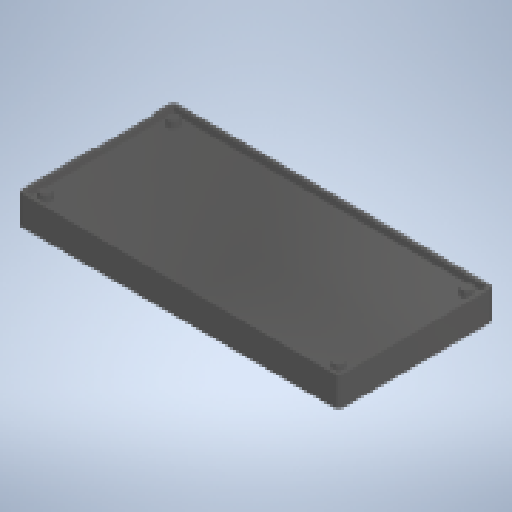
# Autodesk Inventor part: base
Saved by Autodesk Inventor 2025.3 (Build 293356000, 356)
## iProperties
Created: 2025-05-23
Part Number: base
Material: Generic
Document SubType Name: Modeling
Designer: Yuhsuan Chen
Density: 1 g/cm^3
Appearance: Default
Author: Yuhsuan Chen
Autodesk Inventor part; units mm, degrees
ref_plane "YZ Plane" through (0, 0, 0) normal (1, 0, 0) x (0, 1, 0)
ref_plane "XZ Plane" through (0, 0, 0) normal (0, 1, 0) x (-1, 0, 0)
ref_plane "XY Plane" through (0, 0, 0) normal (0, 0, 1) x (1, 0, 0)
sketch "Sketch1" plane through (0, 0, 0) normal (0, 1, 0) x (-1, 0, 0)
  line L0 (0, 20) -> (-92, 20)
  line L1 (-92, 20) -> (-92, -20)
  line L2 (-92, -20) -> (0, -20)
  line L3 (0, -20) -> (0, 20)
  line L4 (-46, 20) -> (-46, -20) construction
  line L5 (0, 0) -> (-92, 0) construction
  line L6 (0.15, 20.15) -> (-92.15, 20.15)
  line L7 (-92.15, 20.15) -> (-92.15, -20.15)
  line L8 (-92.15, -20.15) -> (0.15, -20.15)
  line L9 (0.15, -20.15) -> (0.15, 20.15)
  dimension "d0" = 40
  dimension "d1" = 92
  dimension "d19" = 0.15
  constraints: 20 end point, 4 midpoint, 4 parallel, 2 coincident, 2 perpendicular, 1 horizontal, 3 other
  measures "d0" distance of L2.end L0.start
  measures "d1" distance of L0.start L0.end
  measures "d19" distance between parallel lines of L3 L9
extrude "Extrusion1" add sketch "Sketch1" along normal blind 0.7 contours L3 L2 L1 L0 | L9 L8 L7 L6
sketch "Sketch2" plane through (0, 0.7, 0) normal (0, 1, 0) x (1, 0, 0)
  line L0 (92.15, -20.15) -> (92.15, 20.15) projected
  line L1 (92.15, 20.15) -> (-0.15, 20.15) projected
  line L2 (-0.15, 20.15) -> (-0.15, -20.15) projected
  line L3 (-0.15, -20.15) -> (92.15, -20.15) projected
  line L4 (1.05, -18.95) -> (1.05, 18.95)
  line L5 (1.05, 18.95) -> (90.95, 18.95)
  line L6 (90.95, 18.95) -> (90.95, -18.95)
  line L7 (90.95, -18.95) -> (1.05, -18.95)
  dimension "d20" = 1.2
  constraints: 8 end point, 3 other
  measures "d20" distance between parallel lines of L2 L4
extrude "Extrusion2" add sketch "Sketch2" along normal blind 5.5
sketch "Sketch4" plane through (0, 0, 0) normal (0, 1, 0) x (1, 0, 0)
  line L0 (1.05, -18.95) -> (90.95, -18.95) projected
  line L1 (90.95, -18.95) -> (90.95, 18.95) projected
  line L2 (90.95, 18.95) -> (1.05, 18.95) projected
  line L3 (1.05, 18.95) -> (1.05, -18.95) projected
  line L4 (92.15, 20.15) -> (-0.15, 20.15) projected
  line L5 (-0.15, 20.15) -> (-0.15, -20.15) projected
  line L6 (-0.15, -20.15) -> (92.15, -20.15) projected
  line L7 (92.15, -20.15) -> (92.15, 20.15) projected
  line L8 (1.05, -18.95) -> (1.05, 18.95) projected
  line L9 (1.05, 18.95) -> (90.95, 18.95) projected
  line L10 (90.95, 18.95) -> (90.95, -18.95) projected
  line L11 (90.95, -18.95) -> (1.05, -18.95) projected
  circle A0 centre (2.55, -17.45) radius 1.5
  circle A1 centre (2.55, 17.45) radius 1.5
  circle A2 centre (89.45, 17.45) radius 1.5
  line L12 (-1.15, -21.15) -> (-1.15, 21.15)
  line L13 (-1.15, 21.15) -> (93.15, 21.15)
  line L14 (93.15, 21.15) -> (93.15, -21.15)
  line L15 (93.15, -21.15) -> (-1.15, -21.15)
  line L16 (-0.15, 20.15) -> (-1.15, 20.15)
  line L17 (-0.15, -20.15) -> (-1.15, -20.15)
  line L18 (2.55, -17.45) -> (1.05, -17.45)
  line L19 (2.55, -17.45) -> (2.55, -18.95)
  line L20 (2.55, 17.45) -> (2.55, 18.95)
  line L21 (2.55, 17.45) -> (1.05, 17.45)
  line L22 (89.45, 17.45) -> (89.45, 18.95)
  line L23 (89.45, 17.45) -> (90.95, 17.45)
  circle A3 centre (2.55, -17.55) radius 1.6 projected
  point P0 (0, 0)
  dimension "d21" = 3
  dimension "d22" = 3
  dimension "d24" = 3
  dimension "d25" = 2.7
  dimension "d26" = 2.7
  dimension "d28" = 2.7
  dimension "d29" = 1
  constraints: 24 end point, 10 point on line, 5 perpendicular, 3 centre point, 1 horizontal alignment, 1 vertical alignment, 3 other
  measures "d21" diameter of A0
  measures "d22" diameter of A1
  measures "d24" diameter of A2
  measures "d25" distance from line of L6 L18.start
  measures "d26" distance from line of L5 L18.start
  measures "d28" distance from line of L4 L20.start
  measures "d29" distance between parallel lines of L5 L12
extrude "Extrusion3" add sketch "Sketch4" along normal blind 8 contours L19 L18 A0 | A0 L18 L19 | L21 L20 A1 | A1 L20 L21 | L23 L22 A2 | A2 L22 L23 | L4 L16 L12 L13 L14 L15 L17 L6 L7 | L5 L17 L12 L16
sketch "Sketch7" plane through (0, 8, 0) normal (0, 1, 0) x (1, 0, 0)
  line L0 (0.05, 14.425) -> (6.05, 14.425) projected
  line L1 (0.05, 0.525) -> (6.05, 0.525) projected
  line L2 (-1.15, 21.15) -> (-1.15, -21.15) projected
  line L3 (-1.15, -21.15) -> (93.15, -21.15) projected
  line L4 (93.15, -21.15) -> (93.15, 21.15) projected
  line L5 (93.15, 21.15) -> (-1.15, 21.15) projected
  line L6 (-0.15, 20.15) -> (92.15, 20.15) projected
  line L7 (92.15, 20.15) -> (92.15, -20.15) projected
  line L8 (92.15, -20.15) -> (-0.15, -20.15) projected
  line L9 (-0.15, -20.15) -> (-0.15, 20.15) projected
  line L10 (-0.15, 20.15) -> (-0.15, -20.15) projected
  line L11 (-1.15, 21.15) -> (-1.15, -21.15) projected
  line L12 (-0.15, 15.425) -> (-1.15, 15.425)
  line L13 (-1.15, 15.425) -> (-1.15, -0.475)
  line L14 (-1.15, -0.475) -> (-0.15, -0.475)
  line L15 (-0.15, -0.475) -> (-0.15, 15.425)
  point P0 (0, 0)
  point P1 (-0.15, -0.475)
  point P2 (-1.15, 15.425)
  dimension "d32" = 1
  dimension "d33" = 1
  constraints: 8 end point, 2 parallel, 2 point on line, 1 horizontal, 1 perpendicular
  measures "d32" distance from line of L14.end L1
  measures "d33" distance from line of L0 L12.start
extrude "Extrusion4" cut sketch "Sketch7" against normal blind 0.4 contours L12 L9 L14 L2
sketch "Sketch8" plane through (0, 0.7, 0) normal (0, 1, 0) x (1, 0, 0)
  circle A0 centre (55.0598, -12.05) radius 4.4577 projected
  circle A1 centre (60.1398, -17.13) radius 0.9906 projected
  circle A2 centre (49.9798, -6.97) radius 0.9906 projected
  circle A3 centre (49.9798, -6.97) radius 0.8406
  circle A4 centre (60.1398, -17.13) radius 0.8406
  point P0 (0, 0)
  dimension "d37" = 0.15
  dimension "d38" = 0.15
  constraints: 2 centre point
  measures "d37" radial gap between concentric circles of A2 A3
  measures "d38" radial gap between concentric circles of A1 A4
extrude "Extrusion5" [suppressed]
sketch "Sketch9" plane through (0, 0.7, 0) normal (0, 1, 0) x (1, 0, 0)
  arc A0 (1.05, 17.45) -> (2.55, 18.95) centre (2.55, 17.45) ccw projected
  arc A1 (89.45, 18.95) -> (90.95, 17.45) centre (89.45, 17.45) ccw projected
  arc A2 (1.05, -17.45) -> (2.55, -18.95) centre (2.55, -17.45) ccw projected
  line L0 (90.95, 18.95) -> (89.45, 18.95) projected
  line L1 (1.05, 18.95) -> (1.05, 17.45) projected
  circle A3 centre (2.55, 17.45) radius 1.5 projected
  circle A4 centre (2.55, -17.45) radius 1.5 projected
  circle A5 centre (89.45, -17.45) radius 1.5 projected
  circle A6 centre (89.45, 17.45) radius 1.5 projected
  line L2 (2.55, 17.45) -> (1.05, 17.45)
  line L3 (2.55, 17.45) -> (2.55, 18.95)
  line L4 (89.45, 17.45) -> (89.45, 18.95)
  line L5 (89.45, 17.45) -> (90.95, 17.45)
  line L6 (89.45, -17.45) -> (89.45, -18.95)
  line L7 (89.45, -17.45) -> (90.95, -17.45)
  line L8 (2.55, -17.45) -> (1.05, -17.45)
  line L9 (2.55, -17.45) -> (2.55, -18.95)
  line L10 (1.05, 17.45) -> (1.05, -17.45) projected
  arc A7 (2.55, -18.95) -> (1.05, -17.45) centre (2.55, -17.45) ccw projected
  line L11 (2.55, -18.95) -> (90.95, -18.95) projected
  line L12 (90.95, -18.95) -> (90.95, 17.45) projected
  line L13 (89.45, 18.95) -> (2.55, 18.95) projected
  arc A8 (2.55, 18.95) -> (1.05, 17.45) centre (2.55, 17.45) ccw projected
  line L14 (2.55, 18.95) -> (1.05, 18.95) projected
  arc A9 (90.95, 17.45) -> (89.45, 18.95) centre (89.45, 17.45) ccw projected
  line L15 (90.95, 17.45) -> (90.95, 18.95) projected
  line L16 (1.05, -17.45) -> (1.05, -18.95) projected
  line L17 (1.05, -18.95) -> (2.55, -18.95) projected
  point P0 (0, 0)
  point P1 (90.95, 17.45)
  point P2 (89.45, 18.95)
  point P3 (2.55, 18.95)
  point P4 (1.05, 17.45)
  point P5 (2.55, -18.95)
  point P6 (1.05, -17.45)
  constraints: 16 end point, 6 point on line, 3 perpendicular
extrude "Extrusion6" add sketch "Sketch9" along normal up to surface (5.5 mm away) contours L1 L14 A3 | A0 L13 A1 L12 A5 L11 A4 L10 | L8 L9 A2 | A4 L9 L8 | A2 L17 L16 | L0 L15 A6 | L6 L7 A5 | A5 L7 L6 | A5 L12 L11
fillet "Fillet1" radius 1 4 edges at (-1.15, 4, 21.15) (93.15, 4, 21.15) (93.15, 4, -21.15) (-1.15, 4, -21.15)
equation "\"d22\" = d21"
equation "\"d24\" = d21"
equation "\"d26\" = d25"
equation "\"d28\" = d25"
equation "\"d33\" = d32"
body "Solid1"
